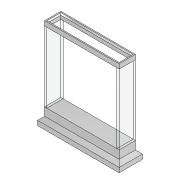
# Autodesk Inventor part: Box
Saved by Autodesk Inventor 2021 (Build 250183000, 183)
## iProperties
Created: 2021-04-01
Part Number: Box
Material: Generic
Document SubType Name: Modeling
Designer: Tran Duc Viet
Mass: 2471.33 g
Surface Area: 2617.1 cm^2
Volume: 2471.33 cm^3
Density: 1 g/cm^3
Appearance: Default
Author: Tran Duc Viet
Autodesk Inventor part; units mm, degrees
ref_plane "YZ Plane" through (0, 0, 0) normal (1, 0, 0) x (0, 1, 0)
ref_plane "XZ Plane" through (0, 0, 0) normal (0, 1, 0) x (-1, 0, 0)
ref_plane "XY Plane" through (0, 0, 0) normal (0, 0, 1) x (1, 0, 0)
sketch "Sketch1" plane through (0, 0, 0) normal (0, 1, 0) x (-1, 0, 0)
  line L0 (150, 25) -> (-150, 25)
  line L1 (-150, 25) -> (-150, -25)
  line L2 (-150, -25) -> (150, -25)
  line L3 (150, -25) -> (150, 25)
  line L4 (150, 25) -> (-150, -25) construction
  line L5 (-150, 25) -> (150, -25) construction
  line L6 (160, 35) -> (-160, 35)
  line L7 (-160, 35) -> (-160, -35)
  line L8 (-160, -35) -> (160, -35)
  line L9 (160, -35) -> (160, 35)
  line L10 (160, 35) -> (-160, -35) construction
  line L11 (-160, 35) -> (160, -35) construction
  point P0 (0, 0)
  dimension "d0" = 300
  dimension "d1" = 50
  dimension "d2" = 320
  dimension "d3" = 70
  constraints: 24 end point, 4 midpoint, 4 parallel, 2 horizontal, 2 perpendicular
  measures "d0" distance of L2.end L1.end
  measures "d1" distance of L1.end L0.end
  measures "d2" distance of L8.end L7.end
  measures "d3" distance of L8.end L6.start
extrude "Extrusion1" add sketch "Sketch1" along normal blind 320
ref_plane "Work Plane1" through (0, 300, 0) normal (0, 1, 0) x (1, 0, 0)
sketch "Sketch2" plane through (0, 0, 0) normal (0, -1, 0) x (1, 0, 0)
  line L0 (160, 35) -> (160, -35) projected
  line L1 (-160, -35) -> (160, -35)
  line L2 (160, -35) -> (160, 35)
  line L3 (160, 35) -> (-160, 35)
  line L4 (-160, 35) -> (-160, -35)
  line L5 (-160, -35) -> (160, 35) construction
  line L6 (160, -35) -> (-160, 35) construction
  point P0 (0, 0)
  constraints: 12 end point, 2 midpoint, 2 parallel, 1 horizontal, 1 perpendicular
extrude "Extrusion2" add sketch "Sketch2" along normal blind 50
sketch "Sketch3" plane through (0, -50, 0) normal (0, -1, 0) x (1, 0, 0)
  line L0 (-175, -50) -> (175, -50)
  line L1 (175, -50) -> (175, 50)
  line L2 (175, 50) -> (-175, 50)
  line L3 (-175, 50) -> (-175, -50)
  line L4 (-175, -50) -> (175, 50) construction
  line L5 (175, -50) -> (-175, 50) construction
  point P0 (0, 0)
  dimension "d9" = 350
  dimension "d10" = 100
  constraints: 12 end point, 2 midpoint, 2 parallel, 1 horizontal, 1 perpendicular
  measures "d9" distance of L2.end L1.end
  measures "d10" distance of L1.end L0.end
extrude "Extrusion3" add sketch "Sketch3" along normal blind 20
chamfer "Chamfer1" distance 15 angle 45 4 edges at (0, -50, 35) (-160, -50, 0) (0, -50, -35) (160, -50, 0)
chamfer "Chamfer2" distance 5 angle 45 4 edges at (0, 320, -25) (-150, 320, 0) (0, 320, 25) (150, 320, 0)
split body "Split1" result two bodies by plane through (0, 300, 0) normal (0, 1, 0) first body at (50, 300.5, 31.6667)
ref_plane "Work Plane2" through (0, 0, 0) normal (0, -1, 0) x (1, 0, 0)
split body "Split2" result two bodies by plane through (0, 0, 0) normal (0, -1, 0) bodies 3 first body at (58.3333, -69.5, -16.6667)
sketch "Sketch4" plane through (-160, 300, 35) normal (0, 0, 1) x (1, 0, 0)
  line L0 (10, -300) -> (10, 0) projected
  line L1 (310, -300) -> (310, 0) projected
  line L2 (10, 0) -> (310, 0)
  line L3 (310, 0) -> (310, -300)
  line L4 (310, -300) -> (10, -300)
  line L5 (10, -300) -> (10, 0)
  point P0 (160, -300)
  constraints: 8 end point, 2 parallel, 1 horizontal, 1 perpendicular
extrude "Extrusion4" cut sketch "Sketch4" against normal through all bodies 5
equation "\"d4\" = d2"
